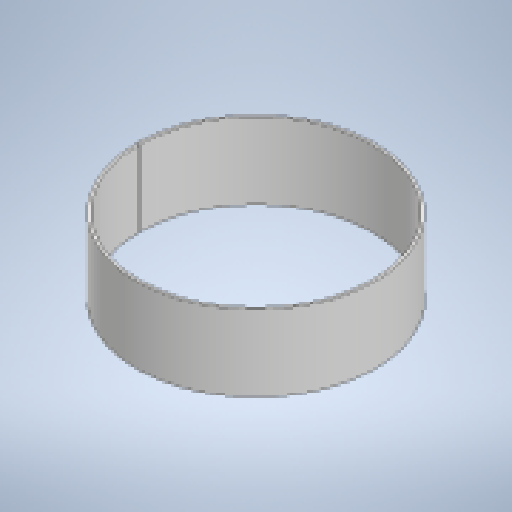
# Autodesk Inventor part: PRS 940-11 accses hatch tube
Saved by Autodesk Inventor 2025.4 (Build 294407000, 407)
## iProperties
Created: 2025-02-12
Part Number: PRS 940-11 accses hatch tube
Material: Generic
Document SubType Name: Sheet Metal
Designer: pokla
Density: 1 g/cm^3
Flat Pattern Width: 165.918 cm
Flat Pattern Length: 17 cm
Flat Pattern Area: 2820.61 cm^2
Sheet Metal Rule: Default_mm
Sheet Metal Width: 1659,180 mm
Sheet Metal Length: 170,000 mm
Sheet Metal Area: 282060,524 mm^2
Appearance: Default
Mass: 1619.32 g
Surface Area: 5634.28 cm^2
Volume: 1619.32 cm^3
Author: pokla
Autodesk Inventor part; units mm, degrees
ref_plane "YZ Plane" through (0, 0, 0) normal (1, 0, 0) x (0, 1, 0)
ref_plane "XZ Plane" through (0, 0, 0) normal (0, 1, 0) x (-1, 0, 0)
ref_plane "XY Plane" through (0, 0, 0) normal (0, 0, 1) x (1, 0, 0)
sketch "Sketch1" plane through (0, 0, 0) normal (0, 1, 0) x (-1, 0, 0)
  line L0 (261.5, 120) -> (261.5, 0)
  line L1 (261.5, 0) -> (267.5, 0)
  line L2 (0, 0) -> (0, 109.131)
  line L3 (261.5, 120) -> (267.5, 120)
  line L4 (267.5, 0) -> (267.5, 120)
  line L5 (267.5, 0) -> (261.5, 0)
  line L6 (261.5, 0) -> (261.5, -50)
  line L7 (261.5, -50) -> (267.5, -50)
  line L8 (267.5, -50) -> (267.5, 0)
  point P0 (264.5, 0)
  point P1 (267.5, 0)
  dimension "d3" = 6
  dimension "d5" = 120
  dimension "d7" = 6
  dimension "d8" = 50
  dimension "d12" = 535
  constraints: 18 end point, 2 horizontal, 2 midpoint, 2 parallel, 2 perpendicular, 2 vertical, 1 horizontal alignment
  measures "d3" distance of L0.end L1.end
  measures "d5" distance between parallel lines of L1 L3
  measures "d7" distance of L6.end L7.end
  measures "d8" distance of L7.end L5.start
  measures "d12" diameter of L4 L2
revolve "Revolution1" add sketch "Sketch1" angle 359.9 about axis through (0, 0, 0) along (0, 0, 1)
sketch "Sketch2" plane through (0, 0, 0) normal (0, 1, 0) x (-1, 0, 0)
  circle A0 centre (0, -476) radius 476
  point P0 (0, 0)
  dimension "d9" = 952
  constraints: 2 vertical alignment, 2 other
extrude "Extrusion1" [suppressed]
equation "\"d5\" = Accsess_hatch_lenght"
equation "\"d7\" = d3"
equation "\"d12\" = Accsess_hatch_diameter"
equation "\"Accsess_hatch_lenght\" = 120"
equation "\"Accsess_hatch_diameter\" = 535"
equation "\"BendRadius\" = Thickness"
equation "\"BendReliefWidth\" = Thickness"
equation "\"BendReliefDepth\" = 0.5 * Thickness"
equation "\"CornerReliefSize\" = 4 * Thickness"
equation "\"MinimumRemnant\" = 2 * Thickness"
equation "\"TransitionRadius\" = BendRadius"
equation "\"JacobiRadiusSize\" = BendRadius"
equation "\"GapSize\" = Thickness"
equation "\"Thickness\" = 6"
body "Solid1"
